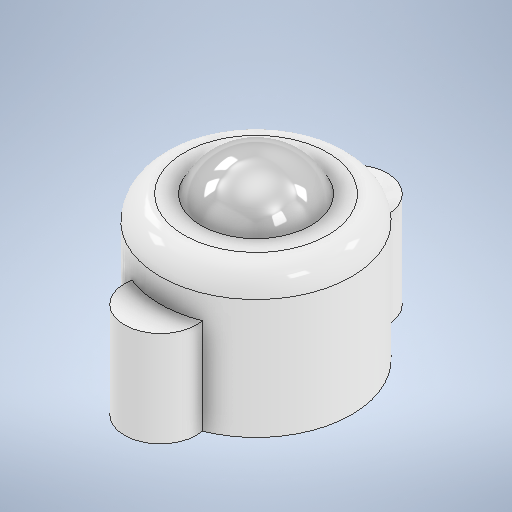
# Autodesk Inventor part: ball_caster
Saved by Autodesk Inventor 2025.2 (Build 292293000, 293)
## iProperties
Created: 2025-06-11
Part Number: ball_caster
Material: Generic
Document SubType Name: Modeling
Designer: cdavi
Density: 1 g/cm^3
Appearance: Default
Author: cdavi
Autodesk Inventor part; units mm, degrees
ref_plane "YZ Plane" through (0, 0, 0) normal (1, 0, 0) x (0, 1, 0)
ref_plane "XZ Plane" through (0, 0, 0) normal (0, 1, 0) x (-1, 0, 0)
ref_plane "XY Plane" through (0, 0, 0) normal (0, 0, 1) x (1, 0, 0)
sketch "Sketch1" plane through (0, 0, 0) normal (0, 1, 0) x (-1, 0, 0)
  circle A0 centre (0, 0) radius 8
  circle A1 centre (0, -8) radius 3
  circle A2 centre (0, 8) radius 3
  point P0 (2.9468, 7.4375)
  point P1 (-2.9468, 7.4375)
  point P2 (-2.9468, -7.4375)
  point P3 (2.9468, -7.4375)
  dimension "d0" = 16
  dimension "d1" = 6
  constraints: 3 centre point, 2 point on circle, 2 vertical alignment, 1 coincident, 1 equal radius
  measures "d0" diameter of A0
  measures "d1" diameter of A1
extrude "Extrusion1" add sketch "Sketch1" along normal blind 12 contours A0 A1 A2 | A2 A0 | A0 A1 picked at (-0.9446, 7.057) picked at (0.9446, -7.057)
extrude "Extrusion2" add sketch "Sketch1" along normal blind 8 contours A0 A2 | A1 A0 picked at (-1.0397, 8.7946) picked at (-1.0397, -8.7946)
fillet "Fillet1" radius 2 1 edges at (-2.9468, 12, 7.4375)
sketch "Sketch2" plane through (0, 12, 0) normal (0, 1, 0) x (1, 0, 0)
  point P0 (0, 0)
sketch "Sketch3" plane through (0, 0, 0) normal (1, 0, 0) x (0, 1, 0)
  circle A0 centre (10, 0) radius 5
  line L0 (12, 6) -> (12, -6) projected
  line L1 (15, 0) -> (5, 0)
  line L2 (0, -7.4375) -> (0, 7.4375) projected
  line L3 (0, -10.4125) -> (0, 10.4125) projected
  line L4 (-4.7416, 0) -> (28.4498, 0) projected
  point P0 (0, 0)
  point P1 (0, 0)
  point P2 (12, 0)
  point P3 (12, -4.5826)
  point P4 (12, 4.5826)
  dimension "d13" = 10
  dimension "d14" = 3
  constraints: 2 end point, 2 point on circle, 1 centre point, 1 coincident, 1 horizontal, 1 horizontal alignment, 1 midpoint, 1 point on line
  measures "d13" diameter of A0
  measures "d14" distance from line of L0 point (15, 0)
revolve "Revolution1" add sketch "Sketch3" angle 360 about axis through (0, -10, 0) along (0, 1, 0) separate body picked at (12.3332, 2.861) contours L1 L0 A0
sketch "Sketch4" plane through (0, 0, 0) normal (0, -1, 0) x (1, 0, 0)
  arc A0 (-2.9468, -7.4375) -> (2.9468, -7.4375) centre (0, -8) ccw projected
  circle A1 centre (0, -8) radius 1
  arc A2 (2.9468, 7.4375) -> (-2.9468, 7.4375) centre (0, 8) ccw projected
  circle A3 centre (0, 8) radius 1
  point P0 (0, 0)
  dimension "d9" = 2
  constraints: 2 centre point, 2 coincident, 1 equal radius
  measures "d9" diameter of A1
extrude "Extrusion3" cut sketch "Sketch4" against normal blind 5 bodies 1
body "Solid1"
body "Solid2"
